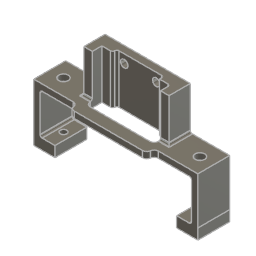
soporte sensor (Autodesk Fusion 360 design; units mm, degrees)
part number: 2026-06-25-21-30-08-012
Autodesk Fusion 360 part; units mm, degrees
note: some values were not read from the file. Chosen so that the rebuilt part matches the saved one: which face or edge a step refers to; which pieces of a blend or face edit are solid. Set by a fixed rule: which sketch regions a step uses.
sketch "Boceto1" plane through (0, 0, 0) normal (0, 1, 0) x (1, 0, 0)
  circle A0 centre (-32, 0) radius 1.525
  circle A1 centre (32, 0) radius 1.525
  line L0 (-35.5, 7.5) -> (-35.5, -7.5)
  line L1 (35.5, 7.5) -> (35.5, -7.5)
  line L2 (-28.5, 7.5) -> (-28.5, -7.5)
  line L3 (28.5, 7.5) -> (28.5, -7.5)
  line L4 (-35.5, 7.5) -> (-28.5, 7.5)
  line L5 (-28.5, -7.5) -> (-35.5, -7.5)
  line L6 (28.5, -7.5) -> (35.5, -7.5)
  line L7 (28.5, 7.5) -> (35.5, 7.5)
  dimension "d1" = 64
  dimension "d2" = 3.05
  dimension "d3" = 3.05
  dimension "d8" = 15
  dimension "d9" = 15
  dimension "d10" = 15
  dimension "d11" = 15
  constraint perpendicular L2 L4
  constraint perpendicular L0 L5
  constraint perpendicular L1 L6
  constraint perpendicular L1 L7
  measures "d1" distance of A0.centre A1.centre
  measures "d2" diameter of A0
  measures "d3" diameter of A1
  measures "d8" distance of L0.start L0.end
  measures "d9" distance of L1.start L1.end
  measures "d10" distance of L2.start L2.end
  measures "d11" distance of L3.start L3.end
extrude "Extruir1" add sketch "Boceto1" along normal blind 4 makes body 1 at (-31.962, 0, 5.5069) makes body 2 at (32.038, 0, 5.5069)
sketch "Boceto2" plane through (0, 0, 0) normal (0, 0, 1) x (1, 0, 0)
  line L0 (-38.5, 4) -> (-38.5, 0)
  line L1 (-35.5, 0) -> (-35.5, 4)
  line L2 (-38.5, 4) -> (-38.5, 19)
  line L3 (-35.5, 4) -> (-35.5, 19)
  line L4 (-38.5, 19) -> (-38.5, 22)
  line L5 (-38.5, 22) -> (35.5, 22)
  line L6 (35.5, 22) -> (38.5, 22)
  line L7 (-35.5, 19) -> (35.5, 19)
  line L8 (35.5, 19) -> (35.5, 4)
  line L9 (35.5, 4) -> (35.5, 0)
  line L10 (38.5, 0) -> (38.5, 22)
  line L11 (-38.5, 0) -> (-38.5, -5)
  line L12 (-38.5, -5) -> (-28.5, -5)
  line L13 (-28.5, -5) -> (-28.5, 0)
  line L14 (-28.5, 0) -> (-35.5, 0)
  line L15 (38.5, 0) -> (38.5, -5)
  line L16 (38.5, -5) -> (28.5, -5)
  line L17 (28.5, -5) -> (28.5, 0)
  line L18 (28.5, 0) -> (35.5, 0)
  line L19 (-35.5, 4) -> (-28.5268, 4)
  line L20 (-28.5268, 4) -> (-28.5, 0)
  line L21 (28.5, 0) -> (28.5, 4.0028)
  line L22 (28.5, 4.0028) -> (35.5, 4)
  dimension "d17" = 3
  dimension "d18" = 15
  dimension "d19" = 15
  dimension "d20" = 3
  dimension "d22" = 3
  dimension "d58" = 5
  dimension "d60" = 5
  constraint parallel L2 L4
  constraint perpendicular L4 L5
  constraint parallel L5 L6
  constraint perpendicular L3 L7
  constraint perpendicular L7 L8
  constraint perpendicular L7 L9
  constraint perpendicular L11 L12
  constraint perpendicular L12 L13
  constraint perpendicular L1 L14
  constraint perpendicular L10 L16
  constraint perpendicular L16 L17
  constraint perpendicular L3 L19
  constraint perpendicular L18 L21
  measures "d17" distance of L1.end L0.start
  measures "d18" distance of L0.start L2.end
  measures "d19" distance of L1.end L3.end
  measures "d20" distance of L2.end L4.end
  measures "d22" distance of L5.end L6.end
  measures "d58" distance of L0.end L11.end
  measures "d60" distance of L10.start L15.end
extrude "Extruir2" add sketch "Boceto2" along normal blind 7.5 and the other way blind 7.5 contours L0 L1 L2 L3 L4 L5 L6 L7 L8 L9 L10 L11 L12 L13 L14 L15 L16 L17 L18 bodies 1 2
fillet "Empalme1" radius 1 2 edges at (-35.5, 4, 0) (35.5, 4, 0) on bodies 1
sketch "Boceto3" plane through (0, 19, 0) normal (0, -1, 0) x (1, 0, 0)
  line L0 (35.5, -7.5) -> (35.5, 7.5)
  line L1 (35.5, 7.5) -> (-35.5, 7.5)
  line L2 (-35.5, 7.5) -> (-35.5, -7.5)
  line L3 (-35.5, -7.5) -> (35.5, -7.5)
  circle A0 centre (-32, 0) radius 2.25
  circle A1 centre (32, 0) radius 2.25
  dimension "d29" = 4.5
  dimension "d30" = 4.5
  measures "d29" diameter of A0
  measures "d30" diameter of A1
hole "Agujero1" at (-32, 19, 0) at (32, 19, 0) direction (0, 1, 0) diameter 3.05 depth 4 tip angle 118 bodies 1
fillet "Empalme2" radius 1 2 edges at (-35.5, 19, 0) (35.5, 19, 0) on bodies 1
sketch "Boceto4" plane through (0, 22, 0) normal (0, 1, 0) x (-1, 0, 0)
  circle A0 centre (32, 0) radius 1.525
  circle A1 centre (-32, 0) radius 1.525
  line L0 (38.5, -7.5) -> (38.5, 7.5)
  line L1 (38.5, 7.5) -> (-38.5, 7.5)
  line L2 (-38.5, 7.5) -> (-38.5, -7.5)
  line L3 (-38.5, -7.5) -> (38.5, -7.5)
  line L4 (0, 0) -> (0, -2)
  line L5 (16, -2) -> (-16, -2)
  line L6 (20, -5.5) -> (-20, -5.5)
  line L7 (20, -2) -> (20, -5.5)
  line L8 (-20, -5.5) -> (-20, -2)
  line L9 (20, -2) -> (20, 2.5)
  line L10 (-20, -2) -> (-20, 2.5)
  line L11 (-20, 2.5) -> (-16, 2.5)
  line L12 (-16, 2.5) -> (-16, -2)
  line L13 (20, 2.5) -> (16, 2.5)
  line L14 (16, 2.5) -> (16, -2)
  line L15 (16, 2.5) -> (16, 3.5)
  line L16 (-16, 3.5) -> (-16, 2.5)
  line L17 (18, 7.5) -> (18, 11)
  line L18 (18, 11) -> (-18, 11)
  line L19 (-18, 11) -> (-18, 7.5)
  line L20 (16, 3.5) -> (16, 5.5)
  line L21 (16, 5.5) -> (-16, 5.5)
  line L22 (-16, 5.5) -> (-16, 3.5)
  point P0 (0, -5.5)
  dimension "d36" = 2
  dimension "d41" = 1
  dimension "d53" = 2
  constraint coincident L4.start origin
  constraint vertical L4
  constraint perpendicular L4 L5
  constraint midpoint L6 P0
  constraint parallel L5 L6
  constraint perpendicular L5 L7
  constraint perpendicular L6 L8
  constraint perpendicular L5 L9
  constraint perpendicular L5 L10
  constraint perpendicular L10 L11
  constraint perpendicular L5 L12
  constraint perpendicular L9 L13
  constraint perpendicular L5 L14
  constraint coincident L4.end L5
  constraint perpendicular L13 L15
  constraint perpendicular L11 L16
  constraint coincident L1 L17.start
  constraint perpendicular L1 L17
  constraint perpendicular L17 L18
  constraint coincident L1 L19.end
  constraint perpendicular L1 L19
  constraint perpendicular L20 L21
  constraint perpendicular L21 L22
  measures "d36" distance of L4.start L4.end
  measures "d41" distance of L13.end L15.end
  measures "d53" distance of L15.end L20.end
extrude "Extruir3" add sketch "Boceto4" along normal blind 20 contours L5 L6 L7 L8 L9 L10 L11 L12 L13 L14 bodies 1
extrude "Extruir4" cut sketch "Boceto4" against normal blind 3 contours L5 L12 L14 L15 L16 L20 L21 L22 bodies 1
fillet "Empalme3" radius 2 5 edges at (0, 22, -5.5) (-20, 22, -1.5) (-18, 22, 2.5) (18, 22, 2.5) (20, 22, -1.5) on bodies 1
sketch "Boceto5" plane through (0, 0, -2) normal (0, 0, 1) x (1, 0, 0)
  line L0 (16, 19) -> (16, 42)
  line L1 (16, 42) -> (-16, 42)
  line L2 (-16, 42) -> (-16, 19)
  line L3 (-16, 19) -> (16, 19)
  circle A0 centre (-7.5, 38) radius 1.75
  circle A1 centre (7.5, 38) radius 1.75
  point P0 (0, 38)
  dimension "d44" = 15
  dimension "d45" = 3.5
  dimension "d46" = 3.5
  measures "d44" distance of A0.centre A1.centre
  measures "d45" diameter of A0
  measures "d46" diameter of A1
extrude "Extruir5" cut sketch "Boceto5" against normal blind 6 contours A0 | A1 bodies 1
delete_face "SuprimirCaras1" 1 faces at (21.8725, 22.004, 0.3734) on bodies 1
delete_face "SuprimirCaras2" 1 faces at (17.3333, 23.8095, 2.5091) on bodies 1
delete_face "SuprimirCaras3" 1 faces at (-19.8617, 22.0137, 4.2659) on bodies 1
delete_face "SuprimirCaras4" 1 faces at (-21.4354, 22.0813, -3.7917) on bodies 1
extrude "Extruir6" add 1 faces at (-2.2869, 28.1234, -5.5) along direction (0, 0, -1) blind 2 on bodies 1 bodies 1
delete_face "SuprimirCaras5" 2 faces at (-6.6667, 23.9996, -6.8333) (6.6667, 22.0023, -7.4045) on bodies 1
fillet "Empalme4" radius 1 4 edges at (-20, 22, -2.5) (-18, 22, 2.5) (18, 22, 2.5) (20, 22, -2.5) on bodies 1
extrude "Extruir7" add sketch "Boceto4" against normal blind 3 contours L1 L17 L18 L19 bodies 1
fillet "Empalme5" radius 2 4 edges at (18, 20.5, 7.5) (18, 20.5, 11) (-18, 20.5, 11) (-18, 20.5, 7.5) on bodies 1
extrude "Extruir8" cut sketch "Boceto2" along normal blind 11 and the other way blind 11 contours L1 L14 L19 L20 | L9 L18 L21 L22 bodies 1
delete_face "SuprimirCaras6" 1 faces at (-28.5, 1.3333, -2.5) on bodies 1
delete_face "SuprimirCaras7" 1 faces at (-35.1901, 4.2763, -2.5) on bodies 1
delete_face "SuprimirCaras8" 1 faces at (34.621, 4.0073, -2.5) on bodies 1
hole "Agujero2" at (-32, 0, 0) at (32, 0, 0) direction (0, -1, 0) diameter 3.05 depth 5 tip angle 118 bodies 1
fillet "Empalme6" radius 1 2 edges at (-35.5, 0, 0) (35.5, 0, 0) on bodies 1
sketch "Boceto6" plane through (0, 42, 0) normal (0, 1, 0) x (-1, 0, 0)
  line L0 (20, -7.5) -> (20, 2.5)
  line L1 (20, 2.5) -> (16, 2.5)
  line L2 (16, 2.5) -> (16, -2)
  line L3 (16, -2) -> (-16, -2)
  line L4 (-16, -2) -> (-16, 2.5)
  line L5 (-16, 2.5) -> (-20, 2.5)
  line L6 (-20, 2.5) -> (-20, -7.5)
  line L7 (-20, -7.5) -> (20, -7.5)
  line L8 (11, -2) -> (-11, -2)
  line L9 (11, -2) -> (11, -4)
  line L10 (11, -4) -> (-11, -4)
  line L11 (-11, -4) -> (-11, -2)
  point P0 (0, -2)
  dimension "d70" = 22
  dimension "d71" = 2
  constraint midpoint L8 P0
  constraint coincident L3 P0
  constraint parallel L3 L8
  constraint perpendicular L3 L9
  constraint perpendicular L9 L10
  constraint perpendicular L3 L11
  measures "d70" distance of L8.start L8.end
  measures "d71" distance of L8.start L9.end
extrude "Extruir9" cut sketch "Boceto6" against normal blind 24 contours L3 L8 L9 L10 L11 bodies 1
fillet "Empalme7" radius 1 4 edges at (-11, 30.5, -4) (-11, 30.5, -2) (11, 30.5, -4) (16, 30.5, -2) on bodies 1
fillet "Empalme8" radius 2 2 edges at (-16, 20.5, 5.5) (16, 20.5, 5.5) on bodies 1
extrude "Extruir10" cut sketch "Boceto3" against normal blind 7 contours A0 | A1 bodies 1
